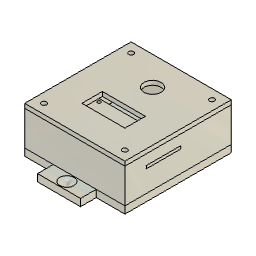
display_internalbtn_holder (Autodesk Fusion 360 design; units mm, degrees)
Autodesk Fusion 360 part; units mm, degrees
sketch "Sketch1" plane through (0, 0, 0) normal (0, 0, 1) x (1, 0, 0)
  line L0 (0, 0) -> (42, 0)
  line L1 (42, 0) -> (42, 24)
  line L2 (42, 24) -> (0, 24)
  line L3 (0, 24) -> (0, 0)
  dimension "d1" = 42
  dimension "d2" = 24
  constraint horizontal L0
  constraint vertical L1
  constraint horizontal L2
  constraint vertical L3
  constraint coincident L0.start L3.end
  measures "d1" distance of L0.start L0.end
  measures "d2" distance of L0.start L2.end
extrude "Extrude1" add sketch "Sketch1" along normal blind 1.6 makes body 1
copy_body "Body->Comp1" bodies 1 removing the originals makes body 2 in component "PCB"
sketch "Sketch2" plane through (0, 0, 1.6) normal (0, 0, 1) x (-1, 0, 0)
  line L0 (0, -24) -> (0, 0)
  line L1 (0, 0) -> (-42, 0)
  line L2 (-42, 0) -> (-42, -24)
  line L3 (-42, -24) -> (0, -24)
  line L4 (-42, 0) -> (-39.9, 0)
  line L5 (-39.9, 0) -> (-39.9, -2.1)
  circle A0 centre (-39.9, -2.1) radius 1.1
  line L6 (-21, 0) -> (-21, -24)
  line L7 (-42, -12) -> (0, -12)
  circle A1 centre (-39.9, -21.9) radius 1.1
  circle A2 centre (-2.1, -21.9) radius 1.1
  circle A3 centre (-2.1, -2.1) radius 1.1
  dimension "d5" = 2.1
  dimension "d6" = 2.1
  dimension "d7" = 2.2
  constraint coincident L1.end L2.start
  constraint perpendicular L2 L4
  constraint perpendicular L4 L5
  constraint coincident L5.end A0.centre
  constraint midpoint L1 L6.start
  constraint midpoint L3 L6.end
  constraint midpoint L2 L7.start
  constraint midpoint L0 L7.end
  constraint symmetric A0 L7 A1
  constraint symmetric A0 L6 A3
  constraint symmetric L6 A1 A2
  measures "d5" distance of L1.end L4.end
  measures "d6" distance of L4.end L5.end
  measures "d7" diameter of A0
extrude "Extrude1'" cut sketch "Sketch2" against normal blind 5 contours A0 | A1 | A2 | A3 bodies 2 in component "PCB"
sketch "Sketch3" plane through (0, 0, 1.6) normal (0, 0, 1) x (-1, 0, 0)
  circle A0 centre (-2.1, -2.1) radius 1.1
  circle A1 centre (-2.1, -21.9) radius 1.1
  circle A2 centre (-39.9, -2.1) radius 1.1
  circle A3 centre (-39.9, -21.9) radius 1.1
  line L0 (0, -24) -> (0, 0)
  line L1 (0, 0) -> (-42, 0)
  line L2 (-42, 0) -> (-42, -24)
  line L3 (-42, -24) -> (0, -24)
  line L4 (-21, 0) -> (-21, -5)
  line L5 (0, -12) -> (-7, -12)
  line L6 (-42, -12) -> (-37, -12)
  line L7 (-21, -24) -> (-21, -19.3)
  line L8 (-7, -12) -> (-7, -24)
  line L9 (-7, -12) -> (-7, 0)
  line L10 (-21, -5) -> (0, -5)
  line L11 (-21, -5) -> (-42, -5)
  line L12 (-37, -12) -> (-37, 0)
  line L13 (-37, -12) -> (-37, -24)
  line L14 (-21, -19.3) -> (-42, -19.3)
  line L15 (-21, -19.3) -> (0, -19.3)
  dimension "d10" = 5
  dimension "d11" = 7
  dimension "d12" = 5
  dimension "d13" = 4.7
  constraint midpoint L1 L4.start
  constraint perpendicular L1 L4
  constraint midpoint L0 L5.start
  constraint perpendicular L0 L5
  constraint midpoint L2 L6.start
  constraint perpendicular L2 L6
  constraint midpoint L3 L7.start
  constraint perpendicular L3 L7
  constraint coincident L3 L8.end
  constraint perpendicular L3 L8
  constraint coincident L1 L9.end
  constraint perpendicular L1 L9
  constraint coincident L0 L10.end
  constraint perpendicular L0 L10
  constraint coincident L2 L11.end
  constraint perpendicular L2 L11
  constraint coincident L1 L12.end
  constraint perpendicular L1 L12
  constraint coincident L3 L13.end
  constraint perpendicular L3 L13
  constraint coincident L2 L14.end
  constraint perpendicular L2 L14
  constraint coincident L0 L15.end
  constraint perpendicular L0 L15
  measures "d10" distance of L4.start L4.end
  measures "d11" distance of L5.start L5.end
  measures "d12" distance of L6.start L6.end
  measures "d13" distance of L7.start L7.end
extrude "Extrude1''" add sketch "Sketch3" along normal blind 7.5 separate body contours L8 L9 L10 L11 L12 L13 L14 L15 makes body 3 in component "Display"
sketch "Sketch4" plane through (0, 0, 1.6) normal (0, 0, 1) x (-1, 0, 0)
  circle A0 centre (-2.1, -2.1) radius 1.1
  circle A1 centre (-2.1, -21.9) radius 1.1
  circle A2 centre (-39.9, -2.1) radius 1.1
  circle A3 centre (-39.9, -21.9) radius 1.1
  line L0 (0, -24) -> (0, 0)
  line L1 (0, 0) -> (-42, 0)
  line L2 (-42, 0) -> (-42, -24)
  line L3 (-42, -24) -> (0, -24)
  line L4 (-42, -12) -> (-40.6, -12)
  line L5 (-40.6, -12) -> (-40.6, -16.9)
  line L6 (-40.6, -12) -> (-40.6, -7.1)
  line L7 (-40.6, -7.1) -> (-38.3, -7.1)
  line L8 (-38.3, -7.1) -> (-38.3, -16.9)
  line L9 (-38.3, -16.9) -> (-40.6, -16.9)
  line L10 (-40.6, -16.9) -> (-40.6, -7.1)
  dimension "d16" = 1.4
  dimension "d17" = 4.9
  dimension "d18" = 4.9
  dimension "d19" = 2.3
  dimension "d20" = 9.8
  constraint midpoint L2 L4.start
  constraint perpendicular L2 L4
  constraint perpendicular L4 L5
  constraint perpendicular L4 L6
  constraint horizontal L7
  constraint vertical L8
  constraint horizontal L9
  constraint vertical L10
  measures "d16" distance of L4.start L4.end
  measures "d17" distance of L4.end L5.end
  measures "d18" distance of L4.end L6.end
  measures "d19" distance of L6.end L7.end
  measures "d20" distance of L6.end L5.end
extrude "Extrude1'''" add sketch "Sketch4" along normal blind 2 separate body contours L5 L6 L7 L8 L9 L10 makes body 4 in component "Headers"
sketch "Sketch5" plane through (0, 0, 3.6) normal (0, 0, 1) x (-1, 0, 0)
  line L0 (-40.6, -16.9) -> (-38.3, -16.9)
  line L1 (-38.3, -16.9) -> (-38.3, -7.1)
  line L2 (-38.3, -7.1) -> (-40.6, -7.1)
  line L3 (-40.6, -7.1) -> (-40.6, -16.9)
extrude "Extrude1''''" add sketch "Sketch5" along normal blind 1.55 separate body makes body 5 in component "Pins"
sketch "Sketch6" plane through (0, 0, 5.15) normal (0, 0, 1) x (-1, 0, 0)
  line L0 (-40.6, -7.1) -> (-40.6, -16.9)
  line L1 (-40.6, -16.9) -> (-38.3, -16.9)
  line L2 (-38.3, -16.9) -> (-38.3, -7.1)
  line L3 (-38.3, -7.1) -> (-40.6, -7.1)
  line L4 (-38.3, -7.1) -> (-40.6, -7.1)
  line L5 (-40.6, -7.1) -> (-40.6, -9.55)
  line L6 (-40.6, -9.55) -> (-38.3, -9.55)
  line L7 (-38.3, -9.55) -> (-38.3, -7.1)
  circle A0 centre (-39.45, -8.325) radius 0.35
  line L8 (-40.6, -9.55) -> (-38.3, -9.55)
  circle A1 centre (-39.45, -10.775) radius 0.35
  line L9 (-40.6, -9.55) -> (-40.6, -12)
  line L10 (-40.6, -12) -> (-38.3, -12)
  circle A2 centre (-39.45, -13.225) radius 0.35
  circle A3 centre (-39.45, -15.675) radius 0.35
  line L11 (-39.45, -8.325) -> (-39.1, -8.325)
  line L12 (-39.1, -8.325) -> (-39.1, -8.675)
  line L13 (-39.1, -8.675) -> (-39.45, -8.675)
  line L14 (-39.45, -8.675) -> (-39.45, -8.325)
  line L15 (-39.1, -8.675) -> (-39.8, -8.675)
  line L16 (-39.8, -8.675) -> (-39.8, -7.975)
  line L17 (-39.8, -7.975) -> (-39.1, -7.975)
  line L18 (-39.1, -7.975) -> (-39.1, -8.675)
  line L19 (-39.45, -10.775) -> (-39.8, -10.775)
  line L20 (-39.8, -10.775) -> (-39.8, -10.425)
  line L21 (-39.8, -10.425) -> (-39.45, -10.425)
  line L22 (-39.45, -10.425) -> (-39.45, -10.775)
  line L23 (-39.45, -10.775) -> (-39.1, -10.775)
  line L24 (-39.1, -10.775) -> (-39.1, -11.125)
  line L25 (-39.1, -11.125) -> (-39.45, -11.125)
  line L26 (-39.45, -11.125) -> (-39.45, -10.775)
  line L27 (-39.1, -11.125) -> (-39.8, -11.125)
  line L28 (-39.8, -11.125) -> (-39.8, -10.425)
  line L29 (-39.8, -10.425) -> (-39.1, -10.425)
  line L30 (-39.1, -10.425) -> (-39.1, -11.125)
  line L31 (-39.8, -13.575) -> (-39.1, -13.575)
  line L32 (-39.8, -12.875) -> (-39.8, -13.575)
  line L33 (-39.1, -12.875) -> (-39.8, -12.875)
  line L34 (-39.1, -13.225) -> (-39.1, -12.875)
  line L35 (-39.1, -13.575) -> (-39.1, -12.875)
  line L36 (-39.8, -15.325) -> (-39.8, -16.025)
  line L37 (-39.8, -16.025) -> (-39.1, -16.025)
  line L38 (-39.1, -16.025) -> (-39.1, -15.325)
  line L39 (-39.1, -15.325) -> (-39.8, -15.325)
  dimension "d25" = 2.45
  dimension "d26" = 0.7
  dimension "d27" = 0.35
  dimension "d28" = 0.35
  dimension "d29" = 0.7
  dimension "d30" = 0.7
  dimension "d31" = 0.35
  dimension "d32" = 0.35
  dimension "d33" = 0.35
  dimension "d34" = 0.35
  constraint horizontal L4
  constraint vertical L5
  constraint horizontal L6
  constraint vertical L7
  constraint coincident L2.end L3.start
  constraint symmetric A0 L8 A1
  constraint midpoint L0 L9.end
  constraint perpendicular L6 L9
  constraint midpoint L2 L10.end
  constraint symmetric A0 L10 A3
  constraint symmetric A1 L10 A2
  constraint horizontal L11
  constraint vertical L12
  constraint horizontal L13
  constraint vertical L14
  constraint coincident A0.centre L11.start
  constraint horizontal L15
  constraint vertical L16
  constraint horizontal L17
  constraint vertical L18
  constraint horizontal L19
  constraint vertical L20
  constraint horizontal L21
  constraint vertical L22
  constraint coincident A1.centre L19.start
  constraint horizontal L23
  constraint vertical L24
  constraint horizontal L25
  constraint vertical L26
  constraint horizontal L27
  constraint vertical L28
  constraint horizontal L29
  constraint vertical L30
  constraint symmetric L10 L12.end L38.end
  constraint symmetric L10 L15.end L36.start
  constraint symmetric L10 L16.end L36.end
  constraint symmetric L10 L17.end L37.end
  constraint symmetric L10 L20.end L31.start
  constraint symmetric L10 L23.end L34.start
  constraint symmetric L10 L24.end L33.start
  constraint symmetric L10 L27.end L32.start
  constraint symmetric L10 L29.end L31.end
  measures "d25" distance of L2.end L6.end
  measures "d26" diameter of A0
  measures "d27" distance of A0.centre L11.end
  measures "d28" distance of A0.centre L13.end
  measures "d29" distance of L12.end L15.end
  measures "d30" distance of L12.end L17.end
  measures "d31" distance of A1.centre L19.end
  measures "d32" distance of A1.centre L21.end
  measures "d33" distance of A1.centre L23.end
  measures "d34" distance of A1.centre L25.end
extrude "Extrude2" cut sketch "Sketch6" against normal blind 1.55 bodies 5 makes body 6 at (39.3333, 13.575, 4.1167) makes body 7 at (39.5667, 11.125, 4.1167) makes body 8 at (39.8, 8.4417, 4.6333) in component "Pins"
sketch "Sketch7" plane through (39.8, 0, 0) normal (1, 0, 0) x (0, 1, 0)
  line L0 (8.675, 5.15) -> (7.975, 5.15)
  line L1 (7.975, 5.15) -> (7.975, 3.6)
  line L2 (7.975, 3.6) -> (8.675, 3.6)
  line L3 (8.675, 3.6) -> (8.675, 5.15)
  line L4 (7.975, 5.15) -> (8.675, 5.15)
  line L5 (8.675, 5.15) -> (8.675, 4.45)
  line L6 (8.675, 4.45) -> (7.975, 4.45)
  line L7 (7.975, 4.45) -> (7.975, 5.15)
  dimension "d37" = 0.7
  constraint horizontal L4
  constraint vertical L5
  constraint horizontal L6
  constraint vertical L7
  constraint coincident L0.end L1.start
  measures "d37" distance of L0.end L6.end
extrude "Extrude3" add sketch "Sketch7" along normal blind 6.5 contours L0 L1 L3 L4 L5 L6 L7 bodies 8 in component "Pins"
sketch "Sketch8" plane through (39.8, 0, 0) normal (1, 0, 0) x (0, 1, 0)
  line L0 (11.125, 5.15) -> (10.425, 5.15)
  line L1 (10.425, 5.15) -> (10.425, 3.6)
  line L2 (10.425, 3.6) -> (11.125, 3.6)
  line L3 (11.125, 3.6) -> (11.125, 5.15)
  line L4 (10.425, 5.15) -> (11.125, 5.15)
  line L5 (11.125, 5.15) -> (11.125, 4.45)
  line L6 (11.125, 4.45) -> (10.425, 4.45)
  line L7 (10.425, 4.45) -> (10.425, 5.15)
  dimension "d40" = 0.7
  dimension "d41" = 0.7
  constraint horizontal L4
  constraint vertical L5
  constraint horizontal L6
  constraint vertical L7
  constraint coincident L0.end L1.start
  measures "d40" distance of L0.end L0.start
  measures "d41" distance of L0.end L6.end
extrude "Extrude4" add sketch "Sketch8" along normal blind 6.5 contours L0 L1 L3 L4 L5 L6 L7 bodies 7 in component "Pins"
sketch "Sketch9" plane through (39.8, 0, 0) normal (1, 0, 0) x (0, 1, 0)
  line L0 (13.575, 5.15) -> (12.875, 5.15)
  line L1 (12.875, 5.15) -> (12.875, 3.6)
  line L2 (12.875, 3.6) -> (13.575, 3.6)
  line L3 (13.575, 3.6) -> (13.575, 5.15)
  line L4 (12.875, 5.15) -> (13.575, 5.15)
  line L5 (13.575, 5.15) -> (13.575, 4.45)
  line L6 (13.575, 4.45) -> (12.875, 4.45)
  line L7 (12.875, 4.45) -> (12.875, 5.15)
  dimension "d44" = 0.7
  dimension "d45" = 0.7
  constraint horizontal L4
  constraint vertical L5
  constraint horizontal L6
  constraint vertical L7
  constraint coincident L0.end L1.start
  measures "d44" distance of L0.end L0.start
  measures "d45" distance of L0.end L6.end
extrude "Extrude5" add sketch "Sketch9" along normal blind 6.5 contours L0 L1 L3 L4 L5 L6 L7 bodies 6 in component "Pins"
sketch "Sketch10" plane through (39.8, 0, 0) normal (1, 0, 0) x (0, 1, 0)
  line L0 (16.025, 5.15) -> (15.325, 5.15)
  line L1 (15.325, 5.15) -> (15.325, 3.6)
  line L2 (15.325, 3.6) -> (16.025, 3.6)
  line L3 (16.025, 3.6) -> (16.025, 5.15)
  line L4 (16.025, 5.15) -> (15.325, 5.15)
  line L5 (15.325, 5.15) -> (15.325, 4.45)
  line L6 (15.325, 4.45) -> (16.025, 4.45)
  line L7 (16.025, 4.45) -> (16.025, 5.15)
  dimension "d48" = 0.7
  dimension "d49" = 0.7
  constraint horizontal L4
  constraint vertical L5
  constraint horizontal L6
  constraint vertical L7
  constraint coincident L0.start L3.end
  measures "d48" distance of L0.start L0.end
  measures "d49" distance of L0.start L6.end
extrude "Extrude6" add sketch "Sketch10" along normal blind 6.5 contours L0 L1 L3 L4 L5 L6 L7 bodies 5 in component "Pins"
sketch "Sketch1 (2)" plane through (0, 0, 9.1) normal (0, 0, 1) x (-1, 0, 0) in component "HW-069"
  line L0 (-37, -5) -> (-37, -19.3)
  line L1 (-37, -19.3) -> (-7, -19.3)
  line L2 (-7, -19.3) -> (-7, -5)
  line L3 (-7, -5) -> (-37, -5)
  line L4 (-57, 15) -> (-57, -39.3)
  line L5 (-57, -39.3) -> (13, -39.3)
  line L6 (13, -39.3) -> (13, 15)
  line L7 (13, 15) -> (-57, 15)
  line L8 (13, -39.3) -> (-57, -39.3)
  line L9 (-57, -39.3) -> (-57, -59.3)
  line L10 (-57, -59.3) -> (13, -59.3)
  line L11 (13, -59.3) -> (13, -39.3)
  circle A0 centre (-22, -39.3) radius 6
  dimension "d52" = 20
  dimension "d53" = 20
  dimension "d54" = 12
  constraint horizontal L8
  constraint vertical L9
  constraint horizontal L10
  constraint vertical L11
  constraint midpoint L5 A0.centre
  measures "d53" distance of L5.end L10.end
  measures "d54" diameter of A0
extrude "Extrude1'''''" add sketch "Sketch1 (2)" against normal blind 3 separate body contours L4 L5 L6 L7 L8 A0 | L5 L8 L9 L10 L11 A0 makes body 9 in component "Front Plate"
sketch "Sketch2 (2)" plane through (0, 0, 6.1) normal (0, 0, -1) x (1, 0, 0) in component "HW-069"
  line L0 (7, -5) -> (37, -5)
  line L1 (37, -5) -> (37, -19.3)
  line L2 (37, -19.3) -> (7, -19.3)
  line L3 (7, -19.3) -> (7, -5)
  circle A0 centre (22, -39.3) radius 6
  line L4 (-13, 15) -> (-13, -59.3)
  line L5 (-13, -59.3) -> (57, -59.3)
  line L6 (57, -59.3) -> (57, 15)
  line L7 (57, 15) -> (-13, 15)
  line L8 (54, -56.3) -> (54, 12)
  line L9 (54, 12) -> (-10, 12)
  line L10 (-10, 12) -> (-10, -56.3)
  line L11 (-10, -56.3) -> (54, -56.3)
  dimension "d57" = -3
extrude "Extrude1''''''" add sketch "Sketch2 (2)" along normal blind 24 separate body contours L4 L5 L6 L7 makes body 10 in component "Walls"
sketch "Sketch11" plane through (-10, 0, 0) normal (1, 0, 0) x (0, 1, 0)
  line L0 (56.3, 6.1) -> (-12, 6.1)
  line L1 (-12, 6.1) -> (-12, -17.9)
  line L2 (-12, -17.9) -> (56.3, -17.9)
  line L3 (56.3, -17.9) -> (56.3, 6.1)
  line L4 (0, 0) -> (24, 0)
  line L5 (24, 0) -> (24, 1.6)
  line L6 (24, 1.6) -> (0, 1.6)
  line L7 (0, 1.6) -> (0, 0)
  line L8 (24, 0) -> (0, 0)
  line L9 (0, 0) -> (0, -3)
  line L10 (0, -3) -> (24, -3)
  line L11 (24, -3) -> (24, 0)
  constraint horizontal L8
  constraint vertical L9
  constraint horizontal L10
  constraint vertical L11
  constraint coincident L4.end L5.start
extrude "Extrude1'''''''" add sketch "Sketch11" along normal blind 67 separate body contours L4 L8 L9 L10 L11 makes body 11 in component "HW-069 Support"
extrude "Extrude2'" cut 1 faces at (34.6667, 8, 0) along direction (0, 0, -1) blind 1 on bodies 11 bodies 10 in component "Walls"
extrude "Extrude2''" cut 1 faces at (34.6667, 8, 0) along direction (0, 0, -1) blind 1 on bodies 11 bodies 11 in component "HW-069 Support"
sketch "Sketch12" plane through (0, 0, -1) normal (0, 0, 1) x (-1, 0, 0)
  line L0 (10, -24) -> (10, 0)
  line L1 (10, 0) -> (-57, 0)
  line L2 (-57, 0) -> (-57, -24)
  line L3 (-57, -24) -> (10, -24)
  circle A0 centre (-2.1, -2.1) radius 1.1
  circle A1 centre (-39.9, -2.1) radius 1.1
  circle A2 centre (-39.9, -21.9) radius 1.1
  circle A3 centre (-2.1, -21.9) radius 1.1
  point P0 (-3.2, -21.9)
extrude "Extrude3'" cut sketch "Sketch12" against normal blind 10 contours A0 | A1 | A2 | A3 bodies 11 in component "HW-069 Support"
sketch "Sketch13" plane through (0, 0, 0) normal (0, -1, 0) x (1, 0, 0)
  line L0 (57, -1) -> (-10, -1)
  line L1 (-10, -1) -> (-10, -3)
  line L2 (-10, -3) -> (57, -3)
  line L3 (57, -3) -> (57, -1)
  line L4 (54, 6.1) -> (54, -18)
  line L5 (54, -18) -> (-10, -18)
  line L6 (-10, -18) -> (-10, 6)
  line L7 (-10, 6) -> (54, 6.1)
  line L8 (54, -3) -> (54, -9)
  line L9 (-10, -3) -> (-10, -9)
  line L10 (-10, -9) -> (0.3923, -3)
  line L11 (-10, -9) -> (2, -9) construction
  line L12 (22, -18) -> (22, 6.05)
  line L13 (54, -9) -> (43.6077, -3)
  point P0 (54, 6.1)
  dimension "d68" = 64
  dimension "d70" = 6
  dimension "d71" = 30
  constraint coincident P0 L4.start
  constraint perpendicular L2 L4
  constraint perpendicular L4 L5
  constraint perpendicular L2 L6
  constraint coincident L4 L8.start
  constraint coincident L2 L8.start
  constraint coincident L4 L8.end
  constraint coincident L1.end L2.start
  constraint perpendicular L2 L9
  constraint horizontal L11
  constraint coincident L2 L10.end
  constraint midpoint L5 L12.start
  constraint midpoint L7 L12.end
  constraint symmetric L9.end L12 L8.end
  constraint symmetric L10.end L12 L13.end
  measures "d68" distance of L4.end L5.end
  measures "d70" distance of L1.end L9.end
  measures "d71" angle of L10 L11
extrude "Extrude3''" add sketch "Sketch13" against normal blind 24 contours L2 L4 L8 L13 | L2 L6 L9 L10 bodies 10 in component "Walls"
sketch "Sketch14" plane through (0, 0, -17.9) normal (0, 0, -1) x (1, 0, 0)
  line L0 (54, -56.3) -> (-10, -56.3)
  line L1 (-10, -56.3) -> (-10, 12)
  line L2 (-10, 12) -> (54, 12)
  line L3 (54, 12) -> (54, -56.3)
  line L4 (57, 15) -> (-13, 15)
  line L5 (-13, 15) -> (-13, -59.3)
  line L6 (-13, -59.3) -> (57, -59.3)
  line L7 (57, -59.3) -> (57, 15)
extrude "Extrude1''''''''" add sketch "Sketch14" along normal blind 5 separate body contours L0 L1 L2 L3 | L4 L5 L6 L7 makes body 12 in component "Back"
sketch "Sketch15" plane through (0, 0, 6.1) normal (0, 0, 1) x (-1, 0, 0)
  line L0 (10, -56.3) -> (-54, -56.3)
  line L1 (-54, -56.3) -> (-54, 12)
  line L2 (-54, 12) -> (10, 12)
  line L3 (10, 12) -> (10, -56.3)
  line L4 (13, 15) -> (-57, 15)
  line L5 (-57, 15) -> (-57, -59.3)
  line L6 (-57, -59.3) -> (13, -59.3)
  line L7 (13, -59.3) -> (13, 15)
  line L8 (-54, -56.3) -> (-46.5, -56.3)
  line L9 (-46.5, -56.3) -> (-46.5, -48.8)
  line L10 (-46.5, -48.8) -> (-54, -48.8)
  line L11 (-54, -48.8) -> (-54, -56.3)
  line L12 (10, -56.3) -> (2.5, -56.3)
  line L13 (2.5, -56.3) -> (2.5, -48.8)
  line L14 (2.5, -48.8) -> (10, -48.8)
  line L15 (10, -48.8) -> (10, -56.3)
  line L16 (10, 12) -> (2.5, 12)
  line L17 (2.5, 12) -> (2.5, 4.5)
  line L18 (2.5, 4.5) -> (10, 4.5)
  line L19 (10, 4.5) -> (10, 12)
  line L20 (-54, 12) -> (-46.5, 12)
  line L21 (-46.5, 12) -> (-46.5, 4.5)
  line L22 (-46.5, 4.5) -> (-54, 4.5)
  line L23 (-54, 4.5) -> (-54, 12)
  dimension "d76" = 7.5
  dimension "d77" = 7.5
  dimension "d78" = 7.5
  dimension "d79" = 7.5
  dimension "d80" = 7.5
  dimension "d81" = 7.5
  dimension "d82" = 7.5
  dimension "d83" = 7.5
  constraint horizontal L8
  constraint vertical L9
  constraint horizontal L10
  constraint vertical L11
  constraint coincident L0.end L1.start
  constraint horizontal L12
  constraint vertical L13
  constraint horizontal L14
  constraint vertical L15
  constraint coincident L0.start L3.end
  constraint horizontal L16
  constraint vertical L17
  constraint horizontal L18
  constraint vertical L19
  constraint coincident L2.end L3.start
  constraint horizontal L20
  constraint vertical L21
  constraint horizontal L22
  constraint vertical L23
  constraint coincident L1.end L2.start
  measures "d76" distance of L0.end L8.end
  measures "d77" distance of L0.end L10.end
  measures "d78" distance of L0.start L12.end
  measures "d79" distance of L0.start L14.end
  measures "d80" distance of L2.end L16.end
  measures "d81" distance of L2.end L18.end
  measures "d82" distance of L1.end L20.end
  measures "d83" distance of L1.end L22.end
extrude "Extrude1'''''''''" add sketch "Sketch15" against normal blind 24 separate body contours L0 L3 L12 L13 L14 L15 | L0 L1 L8 L9 L10 L11 | L2 L3 L16 L17 L18 L19 | L1 L2 L20 L21 L22 L23 makes body 13 at (-5, -4.5, -9.9) makes body 14 at (-7.5, 56.3, -9.9) makes body 15 at (51.5, -4.5, -1.9) makes body 16 at (49, 56.3, -9.9) in component "Component"
sketch "Sketch16" plane through (0, 0, 6.1) normal (0, 0, 1) x (-1, 0, 0)
  line L0 (10, -48.8) -> (2.5, -48.8)
  line L1 (2.5, -48.8) -> (2.5, -56.3)
  line L2 (2.5, -56.3) -> (10, -56.3)
  line L3 (10, -56.3) -> (10, -48.8)
  circle A0 centre (6.25, -52.55) radius 1.5
  line L4 (10, -56.3) -> (-54, -56.3)
  line L5 (-54, -56.3) -> (-54, 12)
  line L6 (-54, 12) -> (10, 12)
  line L7 (10, 12) -> (10, -56.3)
  line L8 (13, 15) -> (-57, 15)
  line L9 (-57, 15) -> (-57, -59.3)
  line L10 (-57, -59.3) -> (13, -59.3)
  line L11 (13, -59.3) -> (13, 15)
  line L12 (-22, -56.3) -> (-22, 12)
  line L13 (10, -56.3) -> (10, 12)
  line L14 (10, -22.15) -> (-54, -22.15)
  circle A1 centre (-50.25, -52.55) radius 1.5
  circle A2 centre (-50.25, 8.25) radius 1.5
  circle A3 centre (6.25, 8.25) radius 1.5
  dimension "d86" = 3
  constraint midpoint L4 L12.start
  constraint midpoint L6 L12.end
  constraint coincident L2.end L3.start
  constraint coincident L6.end L7.start
  constraint midpoint L13 L14.start
  constraint midpoint L5 L14.end
  constraint symmetric A0 L12 A1
  constraint symmetric A0 L14 A3
  constraint symmetric L14 A1 A2
  measures "d86" diameter of A0
extrude "Extrude2'''" cut sketch "Sketch16" against normal blind 55 contours A0 | A1 | A2 | A3 bodies 12 in component "Back"
extrude "Extrude2''''" cut sketch "Sketch16" against normal blind 55 contours A0 | A1 | A2 | A3 bodies 13 14 15 16 in component "Component"
sketch "Sketch17" plane through (0, 0, -22.9) normal (0, 0, -1) x (1, 0, 0)
  circle A0 centre (50.25, 8.25) radius 1.5
  circle A1 centre (50.25, -52.55) radius 1.5
  circle A2 centre (-6.25, 8.25) radius 1.5
  circle A3 centre (-6.25, -52.55) radius 1.5
  line L0 (57, -59.3) -> (57, 15)
  line L1 (57, 15) -> (-13, 15)
  line L2 (-13, 15) -> (-13, -59.3)
  line L3 (-13, -59.3) -> (57, -59.3)
  circle A4 centre (-6.25, -52.55) radius 5
  circle A5 centre (-6.25, 8.25) radius 5
  circle A6 centre (50.25, 8.25) radius 5
  circle A7 centre (50.25, -52.55) radius 5
  dimension "d91" = 10
  dimension "d92" = 10
  dimension "d93" = 10
  dimension "d94" = 10
  constraint concentric A3 A4
  constraint concentric A2 A5
  constraint concentric A0 A6
  constraint concentric A1 A7
  measures "d91" diameter of A4
  measures "d92" diameter of A5
  measures "d93" diameter of A6
  measures "d94" diameter of A7
extrude "Extrude3'''" cut sketch "Sketch17" against normal blind 4 contours A4 | A5 | A6 | A7 bodies 12 in component "Back"
sketch "Sketch18" plane through (0, 0, -18.9) normal (0, 0, -1) x (1, 0, 0)
  circle A0 centre (-6.25, 8.25) radius 1.5
  circle A1 centre (-6.25, 8.25) radius 5
  circle A2 centre (-6.25, 8.25) radius 1.75
  line L0 (57, 15) -> (-13, 15)
  line L1 (-13, 15) -> (-13, -59.3)
  line L2 (-13, -22.15) -> (57, -22.15)
  line L3 (22, 15) -> (22, -61)
  circle A3 centre (50.25, 8.25) radius 1.75
  circle A4 centre (-6.25, -52.55) radius 1.75
  circle A5 centre (50.25, -52.55) radius 1.75
  dimension "d97" = 3.5
  dimension "d98" = 70
  dimension "d99" = 76
  constraint concentric A0 A2
  constraint midpoint L1 L2.start
  constraint perpendicular L1 L2
  constraint midpoint L0 L3.start
  constraint perpendicular L0 L3
  constraint symmetric A2 L3 A3
  constraint symmetric A2 L2 A4
  constraint symmetric L2 A3 A5
  measures "d97" diameter of A2
  measures "d98" distance of L2.start L2.end
  measures "d99" distance of L3.start L3.end
extrude "Extrude2'''''" cut sketch "Sketch18" against normal blind 100 contours A0 | A2 | A3 | A4 | A5 bodies 9 in component "Front Plate"
extrude "Extrude4'" cut sketch "Sketch18" against normal blind 100 contours A0 | A2 | A3 | A4 | A5 bodies 12 in component "Back"
extrude "Extrude3''''" cut sketch "Sketch18" against normal blind 100 contours A0 | A2 | A3 | A4 | A5 bodies 13 14 15 16 in component "Component"
sketch "Sketch19" plane through (0, 0, -22.9) normal (0, 0, -1) x (1, 0, 0)
  circle A0 centre (50.25, 8.25) radius 5
  circle A1 centre (-6.25, 8.25) radius 5
  circle A2 centre (50.25, -52.55) radius 5
  circle A3 centre (-6.25, -52.55) radius 5
  line L0 (57, -59.3) -> (57, 15)
  line L1 (57, 15) -> (-13, 15)
  line L2 (-13, 15) -> (-13, -59.3)
  line L3 (-13, -59.3) -> (57, -59.3)
  line L4 (22, -59.3) -> (37, -59.3)
  line L5 (37, -59.3) -> (37, -65.3)
  line L6 (37, -65.3) -> (22, -65.3)
  line L7 (22, -65.3) -> (22, -59.3)
  line L8 (22, -59.3) -> (7, -59.3)
  line L9 (7, -59.3) -> (7, -65.3)
  line L10 (7, -65.3) -> (22, -65.3)
  line L11 (22, -65.3) -> (22, -59.3)
  line L12 (22, 15) -> (7, 15)
  line L13 (7, 15) -> (7, 21)
  line L14 (7, 21) -> (22, 21)
  line L15 (22, 21) -> (22, 15)
  line L16 (22, 21) -> (37, 21)
  line L17 (37, 21) -> (37, 15)
  line L18 (37, 15) -> (22, 15)
  line L19 (22, 15) -> (22, 21)
  dimension "d106" = 15
  dimension "d107" = 6
  dimension "d108" = 6
  dimension "d109" = 15
  dimension "d110" = 6
  dimension "d111" = 15
  dimension "d112" = 6
  constraint horizontal L4
  constraint vertical L5
  constraint horizontal L6
  constraint vertical L7
  constraint midpoint L3 L4.start
  constraint horizontal L8
  constraint vertical L9
  constraint horizontal L10
  constraint vertical L11
  constraint horizontal L12
  constraint vertical L13
  constraint horizontal L14
  constraint vertical L15
  constraint midpoint L1 L12.start
  constraint horizontal L16
  constraint vertical L17
  constraint horizontal L18
  constraint vertical L19
  measures "d106" distance of L4.start L4.end
  measures "d107" distance of L4.start L6.end
  measures "d108" distance of L4.start L6.end
  measures "d109" distance of L12.start L12.end
  measures "d110" distance of L12.start L14.end
  measures "d111" distance of L14.end L16.end
  measures "d112" distance of L14.end L12.start
extrude "Extrude5'" add sketch "Sketch19" against normal blind 5 contours L3 L4 L5 L6 L7 L11 | L1 L15 L16 L17 L18 L19 | L3 L7 L8 L9 L10 L11 | L1 L12 L13 L14 L15 L19 bodies 12 in component "Back"
sketch "Sketch20" plane through (0, 0, -17.9) normal (0, 0, 1) x (-1, 0, 0)
  circle A0 centre (6.25, -52.55) radius 1.75
  circle A1 centre (6.25, 8.25) radius 1.75
  circle A2 centre (-50.25, -52.55) radius 1.75
  circle A3 centre (-50.25, 8.25) radius 1.75
  line L0 (-57, 15) -> (-57, -59.3)
  line L1 (-57, -59.3) -> (-37, -59.3)
  line L2 (-37, -59.3) -> (-37, -65.3)
  line L3 (-37, -65.3) -> (-7, -65.3)
  line L4 (-7, -65.3) -> (-7, -59.3)
  line L5 (-7, -59.3) -> (13, -59.3)
  line L6 (13, -59.3) -> (13, 15)
  line L7 (13, 15) -> (-7, 15)
  line L8 (-7, 15) -> (-7, 21)
  line L9 (-7, 21) -> (-37, 21)
  line L10 (-37, 21) -> (-37, 15)
  line L11 (-37, 15) -> (-57, 15)
extrude "Extrude6'" add 1 faces at (17, -21, -21.2333) along direction (0, -1, 0) blind 5 on bodies 12 bodies 12 in component "Back"
extrude "Extrude7" add 1 faces at (17, 65.3, -21.2333) along direction (0, 1, 0) blind 5 on bodies 12 bodies 12 in component "Back"
sketch "Sketch21" plane through (0, 0, -17.9) normal (0, 0, 1) x (-1, 0, 0)
  circle A0 centre (6.25, -52.55) radius 1.75
  circle A1 centre (6.25, 8.25) radius 1.75
  circle A2 centre (-50.25, -52.55) radius 1.75
  circle A3 centre (-50.25, 8.25) radius 1.75
  line L0 (-57, 15) -> (-57, -59.3)
  line L1 (-57, -59.3) -> (-37, -59.3)
  line L2 (-37, -59.3) -> (-37, -70.3)
  line L3 (-37, -70.3) -> (-7, -70.3)
  line L4 (-7, -70.3) -> (-7, -59.3)
  line L5 (-7, -59.3) -> (13, -59.3)
  line L6 (13, -59.3) -> (13, 15)
  line L7 (13, 15) -> (-7, 15)
  line L8 (-7, 15) -> (-7, 26)
  line L9 (-7, 26) -> (-37, 26)
  line L10 (-37, 26) -> (-37, 15)
  line L11 (-37, 15) -> (-57, 15)
  circle A4 centre (-22, -64.8) radius 1
  circle A5 centre (-22, 20.5) radius 1
  dimension "d119" = 2
  dimension "d120" = 2
  measures "d119" diameter of A4
  measures "d120" diameter of A5
extrude "Extrude8" cut sketch "Sketch21" against normal blind 12 contours A4 | A5 bodies 12 in component "Back"
fillet "Fillet1" radius 4 2 edges at (22.9323, -20.8616, -17.9) (22.9323, 64.4384, -17.9) on bodies 12 in component "Back"
extrude "Extrude4''" add 1 faces at (55, 8, 0) along direction (0, 0, -1) blind 1 on bodies 10 bodies 10 in component "Walls"
sketch "Sketch22" plane through (0, 0, -22.9) normal (0, 0, -1) x (1, 0, 0)
  circle A0 centre (22, -64.8) radius 1
  circle A1 centre (22, 20.5) radius 1
  circle A2 centre (50.25, 8.25) radius 5
  circle A3 centre (-6.25, 8.25) radius 5
  circle A4 centre (50.25, -52.55) radius 5
  circle A5 centre (-6.25, -52.55) radius 5
  line L0 (57, -59.3) -> (57, 15)
  line L1 (57, 15) -> (37, 15)
  line L2 (37, 15) -> (37, 26)
  line L3 (37, 26) -> (7, 26)
  line L4 (7, 26) -> (7, 15)
  line L5 (7, 15) -> (-13, 15)
  line L6 (-13, 15) -> (-13, -59.3)
  line L7 (-13, -59.3) -> (7, -59.3)
  line L8 (7, -59.3) -> (7, -70.3)
  line L9 (7, -70.3) -> (37, -70.3)
  line L10 (37, -70.3) -> (37, -59.3)
  line L11 (37, -59.3) -> (57, -59.3)
  line L12 (22, -70.3) -> (22, 3.5758)
  line L13 (-13, -22.15) -> (57, -22.15)
  circle A6 centre (22, -22.15) radius 12.5
  dimension "d127" = 25
  constraint midpoint L9 L12.start
  constraint perpendicular L9 L12
  constraint midpoint L6 L13.start
  constraint midpoint L0 L13.end
  constraint midpoint L13 A6.centre
  measures "d127" diameter of A6
extrude "Extrude9" cut sketch "Sketch22" against normal blind 5 contours L12 L13 A6 | L12 L13 A6 | L12 L13 A6 | L12 L13 A6 bodies 12 in component "Back"
component "HW-069" placed x (1, 0, 0) y (0, 1, 0) z (0, 0, 1) at (0, 0, 0)
component "Walls" placed x (1, 0, 0) y (0, 1, 0) z (0, 0, 1) at (0, 0, 0)
component "Front Plate" placed x (1, 0, 0) y (0, 1, 0) z (0, 0, 1) at (0, 0, 0)
component "HW-069 Support" placed x (1, 0, 0) y (0, 1, 0) z (0, 0, 1) at (0, 0, 0)
component "Back" placed x (1, 0, 0) y (0, 1, 0) z (0, 0, 1) at (0, 0, 0)
component "Component" placed x (1, 0, 0) y (0, 1, 0) z (0, 0, 1) at (0, 0, 0)
component "Pins" placed x (1, 0, 0) y (0, 1, 0) z (0, 0, 1) at (0, 0, 0) in component "HW-069"
component "Headers" placed x (1, 0, 0) y (0, 1, 0) z (0, 0, 1) at (0, 0, 0) in component "HW-069"
component "PCB" placed x (1, 0, 0) y (0, 1, 0) z (0, 0, 1) at (0, 0, 0) in component "HW-069"
component "Display" placed x (1, 0, 0) y (0, 1, 0) z (0, 0, 1) at (0, 0, 0) in component "HW-069"
equation "d5 = 1 mm + ( 2.2 / 2 ) * 1 mm"
equation "d6 = 1 mm + ( 2.2 / 2 ) * 1 mm"
equation "d17 = ( 9.8 / 2 ) * 1 mm"
equation "d18 = ( 9.8 / 2 ) * 1 mm"
equation "d25 = 9.800 mm / 4"
equation "d27 = ( 0.7 / 2 ) * 1 mm"
equation "d28 = ( 0.7 / 2 ) * 1 mm"
equation "d31 = ( 0.7 / 2 ) * 1 mm"
equation "d32 = ( 0.7 / 2 ) * 1 mm"
equation "d33 = ( 0.7 / 2 ) * 1 mm"
equation "d34 = ( 0.7 / 2 ) * 1 mm"
equation "d68 = 67.000 mm - 3 mm"
